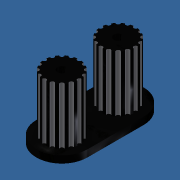
# Autodesk Inventor part: arm-base
Saved by Autodesk Inventor 2015 (Build 190159000, 159)
## iProperties
Created: 2019-02-26
Part Number: arm-base
Material: Generic
Document SubType Name: Modeling
Designer: gabriel
Density: 1 g/cm^3
Appearance: Default
Author: gabriel
Autodesk Inventor part; units mm, degrees
ref_plane "YZ Plane" through (0, 0, 0) normal (1, 0, 0) x (0, 1, 0)
ref_plane "XZ Plane" through (0, 0, 0) normal (0, 1, 0) x (-1, 0, 0)
ref_plane "XY Plane" through (0, 0, 0) normal (0, 0, 1) x (1, 0, 0)
sketch "Sketch12" plane through (0, 0, 0) normal (0, 0, 1) x (1, 0, 0)
  arc A0 (0, -5.7547) -> (0, 5.7547) centre (0, 0) ccw
  arc A1 (-12.7, 5.7547) -> (-12.7, -5.7547) centre (-12.7, 0) ccw
  line L0 (0, 5.7547) -> (-12.7, 5.7547)
  line L1 (0, -5.7547) -> (-12.7, -5.7547)
  dimension "d105" = 5.7547
  dimension "d106" = 12.7
  constraints: 4 end point, 4 point on circle, 4 tangent, 2 centre point, 1 coincident, 1 horizontal, 1 parallel
  measures "d105" radius of A0
  measures "d106" distance of A1.centre point (0, 0)
extrude "Extrusion9" add sketch "Sketch12" along normal blind 1.5875
sketch "Sketch13" plane through (0, 0, 0) normal (0, 0, -1) x (-1, 0, 0)
  arc A0 (0, 5.7547) -> (0, -5.7547) centre (0, 0) ccw projected
  circle A1 centre (0, 0) radius 3.9688
  arc A2 (12.7, -5.7547) -> (12.7, 5.7547) centre (12.7, 0) ccw projected
  circle A3 centre (12.7, 0) radius 3.9688
  dimension "d109" = 7.9375
  dimension "d110" = 7.9375
  constraints: 2 centre point, 2 coincident
  measures "d109" diameter of A1
  measures "d110" diameter of A3
extrude "Extrusion10" add sketch "Sketch13" along normal blind 12.7
sketch "Sketch14" plane through (0, 0, -12.7) normal (0, 0, -1) x (-1, 0, 0)
  circle A0 centre (0, 0) radius 3.9687 projected
  circle A1 centre (0, 3.9687) radius 0.4536
  circle A2 centre (12.7, 0) radius 3.9687 projected
  circle A3 centre (12.7, 3.9687) radius 0.4536
  circle A4 centre (-1.5188, 3.6666) radius 0.4536
  circle A5 centre (-2.8063, 2.8063) radius 0.4536
  circle A6 centre (-3.6666, 1.5188) radius 0.4536
  circle A7 centre (-3.9687, 0) radius 0.4536
  circle A8 centre (-3.6666, -1.5188) radius 0.4536
  circle A9 centre (-2.8063, -2.8063) radius 0.4536
  circle A10 centre (-1.5188, -3.6666) radius 0.4536
  circle A11 centre (0, -3.9687) radius 0.4536
  circle A12 centre (1.5188, -3.6666) radius 0.4536
  circle A13 centre (2.8063, -2.8063) radius 0.4536
  circle A14 centre (3.6666, -1.5188) radius 0.4536
  circle A15 centre (11.1812, 3.6666) radius 0.4536
  circle A16 centre (9.8937, 2.8063) radius 0.4536
  circle A17 centre (9.0334, 1.5188) radius 0.4536
  circle A18 centre (8.7313, 0) radius 0.4536
  circle A19 centre (9.0334, -1.5188) radius 0.4536
  circle A20 centre (9.8937, -2.8063) radius 0.4536
  circle A21 centre (11.1812, -3.6666) radius 0.4536
  circle A22 centre (12.7, -3.9688) radius 0.4536
  circle A23 centre (14.2188, -3.6666) radius 0.4536
  circle A24 centre (15.5063, -2.8063) radius 0.4536
  circle A25 centre (16.3666, -1.5188) radius 0.4536
  circle A26 centre (3.9687, 0) radius 0.4536
  circle A27 centre (3.6666, 1.5188) radius 0.4536
  circle A28 centre (2.8063, 2.8063) radius 0.4536
  circle A29 centre (1.5188, 3.6666) radius 0.4536
  circle A30 centre (16.6688, 0) radius 0.4536
  circle A31 centre (16.3666, 1.5188) radius 0.4536
  circle A32 centre (15.5063, 2.8063) radius 0.4536
  circle A33 centre (14.2188, 3.6666) radius 0.4536
  dimension "d113" = 0.9071
  dimension "d114" = 0.9071
  dimension "d117" = 360
  dimension "d121" = 360
  constraints: 32 centre point, 4 vertical alignment, 68 other
  measures "d113" diameter of A1
  measures "d114" diameter of A3
sketch "Sketch15" plane through (0, 0, -12.7) normal (0, 0, -1) x (-1, 0, 0)
  circle A0 centre (0, 0) radius 0.9922
  arc A1 (12.7, -5.7547) -> (12.7, 5.7547) centre (12.7, 0) ccw projected
  circle A2 centre (12.7, 0) radius 0.9922
  dimension "d125" = 1.9844
  dimension "d126" = 1.9844
  constraints: 2 centre point, 2 coincident
  measures "d125" diameter of A0
  measures "d126" diameter of A2
extrude "Extrusion12" cut sketch "Sketch15" against normal blind 4.7625
extrude "Extrusion14" cut sketch "Sketch14" against normal up to surface (12.7 mm away) contours A0 A26 | A0 A26 | A27 A0 | A0 A27 | A14 A0 | A0 A14 | A28 A0 | A0 A28 | A13 A0 | A0 A13 | A29 A0 | A0 A29 | A12 A0 | A0 A12 | A1 A0 | A0 A1 | A11 A0 | A0 A11 | A4 A0 | A0 A4 | A10 A0 | A0 A10 | A5 A0 | A0 A5 | A9 A0 | A0 A9 | A6 A0 | A0 A6 | A8 A0 | A0 A8 | A7 A0 | A0 A7 | A2 A30 | A2 A30 | A31 A2 | A2 A31 | A25 A2 | A2 A25 | A32 A2 | A2 A32 | A24 A2 | A2 A24 | A33 A2 | A2 A33 | A23 A2 | A2 A23 | A3 A2 | A2 A3 | A22 A2 | A2 A22 | A15 A2 | A2 A15 | A21 A2 | A2 A21 | A16 A2 | A2 A16 | A20 A2 | A2 A20 | A17 A2 | A2 A17 | A19 A2 | A2 A19 | A18 A2 | A2 A18
equation "\"d110\" = d109"
equation "\"d114\" = d113"
equation "\"d126\" = d125"
body "Solid4"
